Autodesk Inventor part; units mm, degrees
(part 3 of 3)
sketch "Sketch78" plane through (-75.2, 2, 54) normal (0, 1, 0) x (1, 0, 0)
  line L0 (56.8805, 54.03) -> (86.8805, 54.03)
  line L1 (86.8805, 54.03) -> (86.8805, 52.03)
  line L2 (86.8805, 52.03) -> (56.8805, 52.03)
  line L3 (56.8805, 52.03) -> (56.8805, 54.03)
  line L4 (-12, -8) -> (162.4, -8) projected
  circle A0 centre (-2.46, 5.26) radius 1.675 projected
  circle A1 centre (7.7, 5.26) radius 1.675 projected
  line L5 (17.3, 78.3) -> (17.3, 97) projected
  line L6 (17.3, 97) -> (-15, 97) projected
  line L7 (-15, 97) -> (-15, 78.3) projected
  line L8 (-15, 78.3) -> (17.3, 78.3) projected
  line L9 (12.24, 7) -> (12.24, 22.5) projected
  line L10 (12.24, 22.5) -> (-7, 22.5) projected
  line L11 (-7, 22.5) -> (-7, 7) projected
  line L12 (-7, 7) -> (12.24, 7) projected
  line L13 (150.4, -4) -> (162.4, -4) projected
  arc A2 (162.4, -4) -> (163.4, -3) centre (162.4, -3) ccw projected
  line L14 (163.4, -3) -> (163.4, -2.2797) projected
  line L15 (163.4, -2.2797) -> (165.4, -2.2797) projected
  line L16 (165.4, -2.2797) -> (165.4, 32.8951) projected
  line L17 (165.4, 32.8951) -> (163.4, 32.8951) projected
  line L18 (163.4, 32.8951) -> (163.4, 48) projected
  line L19 (163.4, 60) -> (163.4, 48) projected
  line L20 (165.4, 60) -> (163.4, 60) projected
  line L21 (165.4, 48) -> (165.4, 60) projected
  line L22 (163.4, 48) -> (165.4, 48) projected
  line L23 (150.4, 0) -> (150.4, -4) projected
  line L24 (130.4, 0) -> (150.4, 0) projected
  line L25 (130.4, -4) -> (130.4, 0) projected
  line L26 (128.4, -4) -> (130.4, -4) projected
  line L27 (128.4, -4) -> (116.4, -4) projected
  line L28 (34, -4) -> (116.4, -4) projected
  line L29 (34, -4) -> (22, -4) projected
  line L30 (20, -4) -> (22, -4) projected
  line L31 (20, 0) -> (20, -4) projected
  line L32 (0, 0) -> (20, 0) projected
  line L33 (0, -4) -> (0, 0) projected
  line L34 (-12, -4) -> (0, -4) projected
  arc A3 (-13, -3) -> (-12, -4) centre (-12, -3) ccw projected
  line L35 (-13, 48) -> (-13, -3) projected
  line L36 (-15, 48) -> (-13, 48) projected
  line L37 (-15, 60) -> (-15, 48) projected
  line L38 (-13, 60) -> (-15, 60) projected
  line L39 (-13, 48) -> (-13, 60) projected
  line L40 (163.4, 60) -> (163.4, 111) projected
  arc A4 (163.4, 111) -> (162.4, 112) centre (162.4, 111) ccw projected
  line L41 (162.4, 112) -> (128.4, 112) projected
  line L42 (128.4, 112) -> (128.4, 114) projected
  line L43 (128.4, 114) -> (116.4, 114) projected
  line L44 (116.4, 114) -> (116.4, 112) projected
  line L45 (116.4, 112) -> (128.4, 112) projected
  line L46 (128.4, -6) -> (128.4, -4) projected
  line L47 (116.4, -6) -> (128.4, -6) projected
  line L48 (116.4, -4) -> (116.4, -6) projected
  line L49 (34, -6) -> (34, -4) projected
  line L50 (22, -6) -> (34, -6) projected
  line L51 (22, -4) -> (22, -6) projected
  line L52 (-13, 74.3) -> (-13, 60) projected
  line L53 (20.3, 74.3) -> (-13, 74.3) projected
  line L54 (20.3, 101) -> (20.3, 74.3) projected
  line L55 (-13, 101) -> (20.3, 101) projected
  line L56 (-13, 111) -> (-13, 101) projected
  arc A5 (-12, 112) -> (-13, 111) centre (-12, 111) ccw projected
  line L57 (22, 112) -> (-12, 112) projected
  line L58 (22, 112) -> (34, 112) projected
  line L59 (34, 112) -> (34, 114) projected
  line L60 (34, 114) -> (22, 114) projected
  line L61 (22, 114) -> (22, 112) projected
  line L62 (116.4, 112) -> (76.7, 112) projected
  line L63 (76.7, 112) -> (76.7, 99.8) projected
  line L64 (76.7, 99.8) -> (58.5, 99.8) projected
  line L65 (58.5, 99.8) -> (58.5, 112) projected
  line L66 (58.5, 112) -> (52.7, 112) projected
  line L67 (52.7, 112) -> (52.7, 99.8) projected
  line L68 (52.7, 99.8) -> (34.5, 99.8) projected
  line L69 (34.5, 99.8) -> (34.5, 112) projected
  line L70 (34.5, 112) -> (34, 112) projected
  line L71 (-13, 74.3) -> (-13, 77.3) projected
  line L72 (-13, 98) -> (-13, 101) projected
  line L73 (150.4, 110.9) -> (150.4, 105.9) projected
  line L74 (150.4, 105.9) -> (130.4, 105.9) projected
  line L75 (130.4, 105.9) -> (130.4, 110.9) projected
  line L76 (130.4, 110.9) -> (150.4, 110.9) projected
  circle A6 centre (124.902, 56.094) radius 1 projected
  circle A7 centre (89.469, 56.094) radius 1 projected
  circle A8 centre (89.469, 91.502) radius 1 projected
  circle A9 centre (124.902, 91.502) radius 1 projected
  circle A10 centre (104.2, 13.0337) radius 1.5 projected
  circle A11 centre (46.2, 13.0337) radius 1.5 projected
  circle A12 centre (46.2, 36.0337) radius 1.5 projected
  circle A13 centre (104.2, 36.0337) radius 1.5 projected
  circle A14 centre (104.2, 13.0337) radius 3 projected
  circle A15 centre (46.2, 13.0337) radius 3 projected
  circle A16 centre (104.2, 36.0337) radius 3 projected
  circle A17 centre (46.2, 36.0337) radius 3 projected
  line L77 (91.971, 89) -> (91.971, 58.596) projected
  line L78 (91.971, 58.596) -> (102, 58.596) projected
  line L79 (102, 58.596) -> (102, 39.596) projected
  line L80 (102, 39.596) -> (110.4, 39.596) projected
  line L81 (110.4, 39.596) -> (110.4, -1.404) projected
  line L82 (110.4, -1.404) -> (122.4, -1.404) projected
  line L83 (122.4, -1.404) -> (122.4, 56.094) projected
  circle A18 centre (124.902, 56.094) radius 2.502 projected
  line L84 (122.4, 56.094) -> (122.4, 89) projected
  line L85 (122.4, 89) -> (91.971, 89) projected
  circle A19 centre (89.469, 56.094) radius 2.502 projected
  circle A20 centre (124.902, 91.502) radius 2.502 projected
  circle A21 centre (89.469, 91.502) radius 2.502 projected
  line L86 (162.4, 32.95) -> (157.4, 32.95) projected
  line L87 (157.4, 32.95) -> (157.4, 72.95) projected
  line L88 (157.4, 72.95) -> (162.4, 72.95) projected
  line L89 (162.4, 72.95) -> (162.4, 32.95) projected
  line L90 (-12, 72.95) -> (-7, 72.95) projected
  line L91 (-7, 72.95) -> (-7, 32.95) projected
  line L92 (-7, 32.95) -> (-12, 32.95) projected
  line L93 (-12, 32.95) -> (-12, 72.95) projected
  line L94 (20, 110.9) -> (20, 105.9) projected
  line L95 (20, 105.9) -> (0, 105.9) projected
  line L96 (0, 105.9) -> (0, 110.9) projected
  line L97 (0, 110.9) -> (20, 110.9) projected
  line L98 (137.4, 37) -> (137.4, 34) projected
  line L99 (137.4, 34) -> (134.2775, 34) projected
  line L100 (134.2775, 34) -> (134.2775, 37) projected
  line L101 (134.2775, 37) -> (137.4, 37) projected
  line L102 (137.4, 37) -> (140.5225, 37) projected
  line L103 (140.5225, 37) -> (140.5225, 34) projected
  line L104 (140.5225, 34) -> (137.4, 34) projected
  arc A22 (-12, 116) -> (-17, 111) centre (-12, 111) ccw projected
  line L105 (-12, 116) -> (36.4, 116) projected
  line L106 (36.4, 116) -> (36.4, 115.5) projected
  line L107 (36.4, 115.5) -> (37, 115.5) projected
  line L108 (37, 115.5) -> (50.2, 115.5) projected
  line L109 (50.2, 115.5) -> (50.8, 115.5) projected
  line L110 (50.8, 115.5) -> (50.8, 116) projected
  line L111 (50.8, 116) -> (60.4, 116) projected
  line L112 (60.4, 116) -> (60.4, 115.5) projected
  line L113 (60.4, 115.5) -> (61, 115.5) projected
  line L114 (61, 115.5) -> (74.2, 115.5) projected
  line L115 (74.2, 115.5) -> (74.8, 115.5) projected
  line L116 (74.8, 115.5) -> (74.8, 116) projected
  line L117 (74.8, 116) -> (162.4, 116) projected
  arc A23 (167.4, 111) -> (162.4, 116) centre (162.4, 111) ccw projected
  line L118 (167.4, 111) -> (167.4, -3) projected
  arc A24 (162.4, -8) -> (167.4, -3) centre (162.4, -3) ccw projected
  line L119 (162.4, -8) -> (-12, -8) projected
  arc A25 (-17, -3) -> (-12, -8) centre (-12, -3) ccw projected
  line L120 (-17, -3) -> (-17, 111) projected
  line L121 (37, 115.5) -> (37, 102.8) projected
  line L122 (37, 102.8) -> (50.2, 102.8) projected
  line L123 (50.2, 102.8) -> (50.2, 115.5) projected
  line L124 (61, 115.5) -> (61, 102.8) projected
  line L125 (61, 102.8) -> (74.2, 102.8) projected
  line L126 (74.2, 102.8) -> (74.2, 115.5) projected
  line L127 (71.8805, 54.03) -> (75.2121, 53.9999) construction
  point P0 (75.2, 54)
  dimension "d533" = 2
  dimension "d534" = 30
  dimension "d535" = 60.03
  constraints: 10 end point, 2 parallel, 1 horizontal, 1 horizontal alignment, 1 midpoint, 1 perpendicular, 1 point on line
  measures "d533" distance of L0.end L1.end
  measures "d534" distance of L0.start L0.end
  measures "d535" distance between parallel lines of L4 L2
extrude "Extrusion65" cut sketch "Sketch78" against normal through all contours L0 L1 L2 L3
sketch "Sketch79" plane through (-75.2, 2, 54) normal (0, 1, 0) x (1, 0, 0)
  line L0 (24, 22.2413) -> (30.2, 22.2413)
  line L1 (30.2, 22.2413) -> (30.2, 16.0413)
  line L2 (30.2, 16.0413) -> (24, 16.0413)
  line L3 (24, 16.0413) -> (24, 22.2413)
  point P0 (75.2, 54)
  dimension "d538" = 6.2
  dimension "d539" = 6.2
  constraints: 8 end point, 2 parallel, 1 horizontal, 1 perpendicular
  measures "d538" distance of L1.end L2.end
  measures "d539" distance of L0.end L1.end
extrude "Extrusion66" cut sketch "Sketch79" against normal blind 1
sketch "Sketch80" plane through (-75.2, 2, 54) normal (0, 1, 0) x (1, 0, 0)
  circle A0 centre (27.1, 19.1413) radius 1.8
  line L0 (24, 16.0413) -> (24, 22.2413) projected
  line L1 (30.2, 22.2413) -> (30.2, 16.0413) projected
  line L2 (24, 16.0413) -> (30.2, 22.2413) construction
  line L3 (24, 22.2413) -> (30.2, 22.2413) projected
  line L4 (30.2, 16.0413) -> (24, 16.0413) projected
  line L5 (24, 22.2413) -> (30.2, 16.0413) construction
  point P0 (75.2, 54)
  dimension "d542" = 3.6
  constraints: 4 end point, 1 centre point, 1 coincident, 1 midpoint
  measures "d542" diameter of A0
extrude "Extrusion67" cut sketch "Sketch80" against normal through all contours A0
pattern_linear "Rectangular Pattern1" count 3 spacing 14.2 along (0, 0, -1) of "Extrusion66", "Extrusion67"
sketch "Sketch81" plane through (-75.2, 2, 54) normal (0, 1, 0) x (1, 0, 0)
  line L0 (18, 53.3413) -> (20, 53.3413)
  line L1 (20, 53.3413) -> (20, 13.3413)
  line L2 (20, 13.3413) -> (18, 13.3413)
  line L3 (18, 13.3413) -> (18, 53.3413)
  line L4 (24, 50.6413) -> (30.2, 50.6413) projected
  line L5 (30.2, 16.0413) -> (24, 16.0413) projected
  line L6 (24, 16.0413) -> (24, 22.2413) projected
  line L7 (30.2, 30.2413) -> (24, 30.2413) projected
  line L8 (24, 36.4413) -> (30.2, 36.4413) projected
  line L9 (34.2, 53.3413) -> (36.2, 53.3413)
  line L10 (36.2, 53.3413) -> (36.2, 13.3413)
  line L11 (36.2, 13.3413) -> (34.2, 13.3413)
  line L12 (34.2, 13.3413) -> (34.2, 53.3413)
  line L13 (30.2, 22.2413) -> (30.2, 16.0413) projected
  line L14 (18, 13.3413) -> (36.2, 13.3413)
  line L15 (36.2, 13.3413) -> (36.2, 11.3413)
  line L16 (36.2, 11.3413) -> (18, 11.3413)
  line L17 (18, 11.3413) -> (18, 13.3413)
  point P0 (75.2, 54)
  point P1 (20, 13.3413)
  point P2 (36.2, 12.3413)
  point P3 (20, 13.3413)
  point P4 (20, 13.3413)
  dimension "d556" = 40
  dimension "d557" = 16.9
  dimension "d558" = 16.9
  dimension "d562" = 40
  dimension "d563" = 16.9
  dimension "d564" = 2
  dimension "d565" = 4
  dimension "d566" = 4
  dimension "d580" = 2
  dimension "d581" = 2
  constraints: 24 end point, 6 parallel, 3 horizontal, 3 perpendicular, 2 point on line, 1 midpoint
  measures "d556" distance of L2.end L0.start
  measures "d557" distance between parallel lines of L7 L2
  measures "d558" distance between parallel lines of L0 L8
  measures "d562" distance of L9.end L10.end
  measures "d563" distance between parallel lines of L8 L9
  measures "d564" distance of L9.start L9.end
  measures "d565" distance between parallel lines of L1 L6
  measures "d566" distance between parallel lines of L13 L12
  measures "d580" distance between parallel lines of L1 L3
  measures "d581" distance between parallel lines of L16 L14
extrude "Extrusion68" add sketch "Sketch81" along normal blind 7
chamfer "Chamfer18" distance 2 angle 45 3 edges at (-39, 2, 21.6587) (-48.1, 2, 42.6587) (-57.2, 2, 21.6587)
sketch "Sketch85" plane through (-55.2, 2, 40.6587) normal (1, 0, 0) x (0, 0, -1)
  line L0 (40, 2) -> (40, 7) projected
  line L1 (0, 7) -> (40, 7)
  line L2 (40, 7) -> (40, 5)
  line L3 (40, 5) -> (0, 5)
  line L4 (0, 5) -> (0, 7)
  line L5 (40, 7) -> (-2, 7) projected
  line L6 (95.5587, 12.8) -> (95.5587, 14) projected
  line L7 (95.5587, 14) -> (97.5587, 14) projected
  line L8 (97.5587, 14) -> (97.5587, 0) projected
  line L9 (97.5587, 0) -> (98.6587, 0) projected
  line L10 (98.6587, 0) -> (100.6587, 2) projected
  line L11 (100.6587, 2) -> (100.6587, 15) projected
  line L12 (100.6587, 15) -> (102.6587, 15) projected
  line L13 (102.6587, 15) -> (102.6587, -2) projected
  line L14 (102.6587, -2) -> (-21.3413, -2) projected
  line L15 (-21.3413, -2) -> (-21.3413, 15) projected
  line L16 (-21.3413, 15) -> (-19.3413, 15) projected
  line L17 (-19.3413, 15) -> (-19.3413, 2) projected
  line L18 (-19.3413, 2) -> (-18.3413, 1) projected
  line L19 (-18.3413, 1) -> (-17.3413, 0) projected
  line L20 (-17.3413, 0) -> (-13.3413, 0) projected
  line L21 (-13.3413, 0) -> (-4, 0) projected
  line L22 (-4, 0) -> (-2, 2) projected
  line L23 (-2, 2) -> (-2, 7) projected
  line L24 (-2, 7) -> (0, 7) projected
  line L25 (0, 7) -> (0, 0) projected
  line L26 (0, 0) -> (40, 0) projected
  line L27 (40, 0) -> (60.9587, 0) projected
  line L28 (60.9587, 0) -> (61.2587, 0.3) projected
  line L29 (61.2587, 0.3) -> (87.3587, 0.3) projected
  line L30 (87.3587, 0.3) -> (87.6587, 0) projected
  line L31 (87.6587, 0) -> (92.5587, 0) projected
  line L32 (92.5587, 0) -> (97.5587, 0) projected
  line L33 (92.5587, 12.8) -> (95.5587, 12.8) projected
  line L34 (92.5587, 0) -> (92.5587, 12.8) projected
  line L35 (-18.3413, 1) -> (-18.3413, 14) projected
  line L36 (-18.3413, 14) -> (-16.3413, 14) projected
  line L37 (-16.3413, 14) -> (-16.3413, 12.8) projected
  line L38 (-16.3413, 12.8) -> (-13.3413, 12.8) projected
  line L39 (-13.3413, 12.8) -> (-13.3413, 0) projected
  line L40 (0, 7) -> (40, 7) projected
  line L41 (40, 7) -> (40, 0) projected
  point P0 (40.6587, -2)
  point P1 (19, 7)
  point P2 (0, 6)
  dimension "d585" = 2
  constraints: 8 end point, 3 point on line, 2 midpoint, 2 parallel, 1 horizontal, 1 perpendicular
  measures "d585" distance between parallel lines of L1 L3
extrude "Extrusion72" add sketch "Sketch85" along normal blind 2 contours L3 L4 L1 L0
sketch "Sketch86" plane through (-41, 2, 0.6587) normal (-1, 0, 0) x (0, 0, 1)
  line L0 (0, 0) -> (0, 7) projected
  line L1 (40, 0) -> (40, 7) projected
  line L2 (0, 7) -> (40, 7)
  line L3 (40, 7) -> (40, 5)
  line L4 (40, 5) -> (0, 5)
  line L5 (0, 5) -> (0, 7)
  point P0 (-0.6587, -2)
  point P1 (0, 5)
  dimension "d588" = 2
  constraints: 8 end point, 2 parallel, 1 horizontal, 1 perpendicular, 1 point on line
  measures "d588" distance between parallel lines of L2 L4
extrude "Extrusion73" add sketch "Sketch86" along normal blind 2
sketch "Sketch87" plane through (-41, 2, 40.6587) normal (0, 0, -1) x (-1, 0, 0)
  line L0 (16.2, 7) -> (-2, 7) projected
  line L1 (14.2, 0) -> (14.2, 12.8) projected
  line L2 (0, 7) -> (14.2, 7)
  line L3 (14.2, 7) -> (14.2, 5)
  line L4 (14.2, 5) -> (0, 5)
  line L5 (0, 5) -> (0, 7)
  point P0 (-41, -2)
  dimension "d591" = 2
  constraints: 8 end point, 2 parallel, 2 point on line, 1 horizontal, 1 perpendicular
  measures "d591" distance between parallel lines of L0 L4
extrude "Extrusion74" add sketch "Sketch87" along normal blind 2
body "Solid1"
